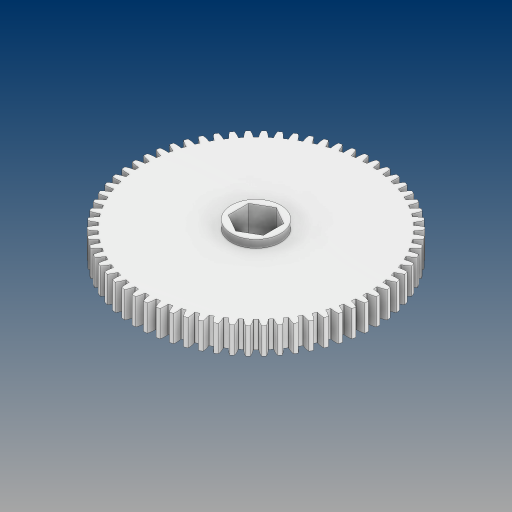
# Autodesk Inventor part: SHOT_1_004_66TGear-24TPulley
Saved by Autodesk Inventor 2024.3 (Build 283343000, 343)
## iProperties
Created: 2024-08-09
Part Number: SHOT_1_004_66TGear-24TPulley
Material: ABS Plastic
Document SubType Name: Modeling
Designer: Kenji
Density: 1.06 g/cm^3
Appearance: Smooth - White
Author: Kenji
Autodesk Inventor part; units mm, degrees
(part 1 of 2)
ref_plane "YZ Plane" through (0, 0, 0) normal (1, 0, 0) x (0, 1, 0)
ref_plane "XZ Plane" through (0, 0, 0) normal (0, 1, 0) x (-1, 0, 0)
ref_plane "XY Plane" through (0, 0, 0) normal (0, 0, 1) x (1, 0, 0)
sketch "Sketch1" plane through (0, 0, 0) normal (0, 1, 0) x (-1, 0, 0)
  circle A0 centre (0, 0) radius 41.91 construction
  line L0 (0, 0) -> (41.91, 0) construction
  line L1 (0, 0) -> (39.2827, 10.1592) construction
  line L2 (39.2827, 10.1592) -> (41.91, 0) construction
  arc A1 (39.2827, 10.1592) -> (37.9956, 14.2362) centre (0, 0) ccw construction
  arc A2 (40.5744, -0.225) -> (39.2827, 10.1592) centre (0, 0) ccw construction
  circle A3 centre (0, 0) radius 43.18
  line L3 (40.3225, 15.447) -> (40.3225, -15.447) construction
  line L4 (40.5744, -0.225) -> (41.91, 0) construction
  line L5 (40.5744, -0.225) -> (40.3225, -0.2901) construction
  line L6 (41.4814, 11.992) -> (38.8764, -18.7919) construction
  line L7 (40.5744, -0.225) -> (40.4457, -0.2469) construction
  line L8 (40.4457, -0.2469) -> (40.3225, -0.2901) construction
  line L9 (41.6879, 11.253) -> (38.5364, -19.4798) construction
  line L10 (40.5744, -0.225) -> (40.5099, -0.2348) construction
  line L11 (40.5099, -0.2348) -> (40.4457, -0.2469) construction
  line L12 (41.1912, 12.9537) -> (39.303, -17.8825) construction
  line L13 (40.5744, -0.225) -> (40.382, -0.2624) construction
  line L14 (40.4457, -0.2469) -> (40.382, -0.2624) construction
  line L15 (40.382, -0.2624) -> (40.3225, -0.2901) construction
  spline S0 degree 4 poles (40.5744, -0.225) (40.5088, -0.2321) (40.4478, -0.2504) (40.3776, -0.2514) (40.3225, -0.2901) knots 0 0 0 0 0 1 1 1 1 1
  line L16 (37.9956, 14.2362) -> (43.1781, 0.4045) construction
  arc A4 (40.3121, -0.9596) -> (40.3225, -0.2901) centre (0, 0) ccw
  line L17 (40.3121, -0.9596) -> (0, 0) construction
  arc A5 (43.1678, -1.0276) -> (43.1781, 0.4045) centre (0, 0) ccw construction
  line L18 (43.1678, -1.0276) -> (40.3121, -0.9596) construction
  arc A6 (43.11, -2.4585) -> (43.1678, -1.0276) centre (0, 0) ccw construction
  spline S1 degree 2 poles (43.1781, 0.4045) (41.9324, -0.0925) (40.5744, -0.225) knots 0 0 0 1 1 1
  spline S2 degree 4 poles (40.5392, -1.7059) (40.4739, -1.6957) (40.4139, -1.6745) (40.3438, -1.6702) (40.2906, -1.6288) knots 0 0 0 0 0 1 1 1 1 1
  arc A7 (40.2906, -1.6288) -> (40.3121, -0.9596) centre (0, 0) ccw
  spline S3 degree 2 poles (43.11, -2.4585) (41.8893, -1.9028) (40.5392, -1.7059) knots 0 0 0 1 1 1
  spline S4 degree 2 poles (42.9441, 4.507) (41.7513, 3.8939) (40.4121, 3.6329) knots 0 0 0 1 1 1
  spline S5 degree 2 poles (43.1484, 1.6505) (41.8805, 2.0876) (40.5178, 2.1553) knots 0 0 0 1 1 1
  spline S6 degree 4 poles (40.5178, 2.1553) (40.4519, 2.1593) (40.39, 2.1747) (40.3199, 2.1723) (40.263, 2.2084) knots 0 0 0 0 0 1 1 1 1 1
  arc A8 (40.263, 2.2084) -> (40.2208, 2.8766) centre (0, 0) ccw
  arc A9 (40.2208, 2.8766) -> (40.1675, 3.5441) centre (0, 0) ccw
  spline S7 degree 4 poles (40.4121, 3.6329) (40.3474, 3.6196) (40.2884, 3.5956) (40.2187, 3.5879) (40.1675, 3.5441) knots 0 0 0 0 0 1 1 1 1 1
  spline S8 degree 2 poles (42.3213, 8.5687) (41.1921, 7.845) (39.8838, 7.4578) knots 0 0 0 1 1 1
  spline S9 degree 2 poles (42.7962, 5.7445) (41.4924, 6.0591) (40.1294, 5.997) knots 0 0 0 1 1 1
  spline S10 degree 4 poles (40.1294, 5.997) (40.0634, 5.9947) (40.0004, 6.0041) (39.9308, 5.9951) (39.8708, 6.0257) knots 0 0 0 0 0 1 1 1 1 1
  arc A10 (39.8708, 6.0257) -> (39.7652, 6.6869) centre (0, 0) ccw
  arc A11 (39.7652, 6.6869) -> (39.6487, 7.3462) centre (0, 0) ccw
  spline S11 degree 4 poles (39.8838, 7.4578) (39.8207, 7.4385) (39.7642, 7.409) (39.6955, 7.3947) (39.6487, 7.3462) knots 0 0 0 0 0 1 1 1 1 1
  spline S12 degree 2 poles (41.3151, 12.5528) (40.2599, 11.725) (38.9943, 11.2153) knots 0 0 0 1 1 1
  spline S13 degree 2 poles (42.0563, 9.7866) (40.7286, 9.9758) (39.3777, 9.7844) knots 0 0 0 1 1 1
  spline S14 degree 4 poles (39.3777, 9.7844) (39.3122, 9.7758) (39.2486, 9.7792) (39.1802, 9.7636) (39.1175, 9.7883) knots 0 0 0 0 0 1 1 1 1 1
  arc A12 (39.1175, 9.7883) -> (38.9496, 10.4365) centre (0, 0) ccw
  arc A13 (38.9496, 10.4365) -> (38.7709, 11.0818) centre (0, 0) ccw
  spline S15 degree 4 poles (38.9943, 11.2153) (38.9333, 11.19) (38.8799, 11.1552) (38.8128, 11.1345) (38.7709, 11.0818) knots 0 0 0 0 0 1 1 1 1 1
  spline S16 degree 2 poles (39.9348, 16.4232) (38.9631, 15.4988) (37.7516, 14.8711) knots 0 0 0 1 1 1
  spline S17 degree 2 poles (40.9356, 13.7399) (39.5959, 13.8021) (38.2693, 13.4832) knots 0 0 0 1 1 1
  spline S18 degree 4 poles (38.2693, 13.4832) (38.2049, 13.4684) (38.1413, 13.4658) (38.0746, 13.4437) (38.0099, 13.4624) knots 0 0 0 0 0 1 1 1 1 1
  arc A14 (38.0099, 13.4624) -> (37.7811, 14.0916) centre (0, 0) ccw
  arc A15 (37.7811, 14.0916) -> (37.5419, 14.717) centre (0, 0) ccw
  spline S19 degree 4 poles (37.7516, 14.8711) (37.6933, 14.8402) (37.6434, 14.8005) (37.5787, 14.7735) (37.5419, 14.717) knots 0 0 0 0 0 1 1 1 1 1
  spline S20 degree 2 poles (38.1929, 20.1449) (37.3134, 19.1323) (36.1671, 18.3923) knots 0 0 0 1 1 1
  spline S21 degree 2 poles (39.4442, 17.5689) (38.1047, 17.5035) (36.8144, 17.0599) knots 0 0 0 1 1 1
  spline S22 degree 4 poles (36.8144, 17.0599) (36.7517, 17.039) (36.6886, 17.0303) (36.6243, 17.0021) (36.5581, 17.0145) knots 0 0 0 0 0 1 1 1 1 1
  arc A16 (36.5581, 17.0145) -> (36.2706, 17.6192) centre (0, 0) ccw
  arc A17 (36.2706, 17.6192) -> (35.973, 18.219) centre (0, 0) ccw
  spline S23 degree 4 poles (36.1671, 18.3923) (36.112, 18.3559) (36.0661, 18.3117) (36.0042, 18.2787) (35.973, 18.219) knots 0 0 0 0 0 1 1 1 1 1
  spline S24 degree 2 poles (36.1051, 23.6841) (35.3258, 22.5926) (34.255, 21.7469) knots 0 0 0 1 1 1
  spline S25 degree 2 poles (37.5956, 21.2388) (36.2683, 21.0463) (35.026, 20.4821) knots 0 0 0 1 1 1
  spline S26 degree 4 poles (35.026, 20.4821) (34.9656, 20.4554) (34.9036, 20.4407) (34.8423, 20.4065) (34.7752, 20.4125) knots 0 0 0 0 0 1 1 1 1 1
  arc A18 (34.7752, 20.4125) -> (34.4315, 20.9871) centre (0, 0) ccw
  arc A19 (34.4315, 20.9871) -> (34.0783, 21.5559) centre (0, 0) ccw
  spline S27 degree 4 poles (34.255, 21.7469) (34.2036, 21.7055) (34.1622, 21.6571) (34.1037, 21.6183) (34.0783, 21.5559) knots 0 0 0 0 0 1 1 1 1 1
  spline S28 degree 2 poles (33.6903, 27.0089) (33.0183, 25.8482) (32.0327, 24.9046) knots 0 0 0 1 1 1
  spline S29 degree 2 poles (35.4065, 24.7163) (34.1035, 24.3985) (32.9205, 23.7188) knots 0 0 0 1 1 1
  spline S30 degree 4 poles (32.9205, 23.7188) (32.8629, 23.6864) (32.8026, 23.6659) (32.7448, 23.626) (32.6774, 23.6257) knots 0 0 0 0 0 1 1 1 1 1
  arc A20 (32.6774, 23.6257) -> (32.2807, 24.165) centre (0, 0) ccw
  arc A21 (32.2807, 24.165) -> (31.875, 24.6977) centre (0, 0) ccw
  spline S31 degree 4 poles (32.0327, 24.9046) (31.9855, 24.8585) (31.9488, 24.8064) (31.8943, 24.7622) (31.875, 24.6977) knots 0 0 0 0 0 1 1 1 1 1
  spline S32 degree 2 poles (30.9703, 30.089) (30.4117, 28.8697) (29.5204, 27.8367) knots 0 0 0 1 1 1
  spline S33 degree 2 poles (32.8967, 27.97) (31.6298, 27.5298) (30.5168, 26.7406) knots 0 0 0 1 1 1
  spline S34 degree 4 poles (30.5168, 26.7406) (30.4625, 26.703) (30.4044, 26.6769) (30.3507, 26.6317) (30.2837, 26.6249) knots 0 0 0 0 0 1 1 1 1 1
  arc A22 (30.2837, 26.6249) -> (29.8375, 27.1241) centre (0, 0) ccw
  arc A23 (29.8375, 27.1241) -> (29.383, 27.6157) centre (0, 0) ccw
  spline S35 degree 4 poles (29.5204, 27.8367) (29.4777, 27.7863) (29.4462, 27.731) (29.3961, 27.6818) (29.383, 27.6157) knots 0 0 0 0 0 1 1 1 1 1
  spline S36 degree 2 poles (27.97, 32.8967) (27.5298, 31.6298) (26.7406, 30.5168) knots 0 0 0 1 1 1
  spline S37 degree 2 poles (30.089, 30.9703) (28.8697, 30.4117) (27.8367, 29.5204) knots 0 0 0 1 1 1
  spline S38 degree 4 poles (27.8367, 29.5204) (27.7863, 29.4777) (27.731, 29.4462) (27.6818, 29.3961) (27.6157, 29.383) knots 0 0 0 0 0 1 1 1 1 1
  arc A24 (27.6157, 29.383) -> (27.1241, 29.8375) centre (0, 0) ccw
  arc A25 (27.1241, 29.8375) -> (26.6249, 30.2837) centre (0, 0) ccw
  spline S39 degree 4 poles (26.7406, 30.5168) (26.703, 30.4625) (26.6769, 30.4044) (26.6317, 30.3507) (26.6249, 30.2837) knots 0 0 0 0 0 1 1 1 1 1
  spline S40 degree 2 poles (24.7163, 35.4065) (24.3985, 34.1035) (23.7188, 32.9205) knots 0 0 0 1 1 1
  spline S41 degree 2 poles (27.0089, 33.6903) (25.8482, 33.0183) (24.9046, 32.0327) knots 0 0 0 1 1 1
  spline S42 degree 4 poles (24.9046, 32.0327) (24.8585, 31.9855) (24.8064, 31.9488) (24.7622, 31.8943) (24.6977, 31.875) knots 0 0 0 0 0 1 1 1 1 1
  arc A26 (24.6977, 31.875) -> (24.165, 32.2807) centre (0, 0) ccw
  arc A27 (24.165, 32.2807) -> (23.6257, 32.6774) centre (0, 0) ccw
  spline S43 degree 4 poles (23.7188, 32.9205) (23.6864, 32.8629) (23.6659, 32.8026) (23.626, 32.7448) (23.6257, 32.6774) knots 0 0 0 0 0 1 1 1 1 1
  spline S44 degree 2 poles (21.2388, 37.5956) (21.0463, 36.2683) (20.4821, 35.026) knots 0 0 0 1 1 1
  spline S45 degree 2 poles (23.6841, 36.1051) (22.5926, 35.3258) (21.7469, 34.255) knots 0 0 0 1 1 1
  spline S46 degree 4 poles (21.7469, 34.255) (21.7055, 34.2036) (21.6571, 34.1622) (21.6183, 34.1037) (21.5559, 34.0783) knots 0 0 0 0 0 1 1 1 1 1
  arc A28 (21.5559, 34.0783) -> (20.9871, 34.4315) centre (0, 0) ccw
  arc A29 (20.9871, 34.4315) -> (20.4125, 34.7752) centre (0, 0) ccw
  spline S47 degree 4 poles (20.4821, 35.026) (20.4554, 34.9656) (20.4407, 34.9036) (20.4065, 34.8423) (20.4125, 34.7752) knots 0 0 0 0 0 1 1 1 1 1
  spline S48 degree 2 poles (17.5689, 39.4442) (17.5035, 38.1047) (17.0599, 36.8144) knots 0 0 0 1 1 1
  spline S49 degree 2 poles (20.1449, 38.1929) (19.1323, 37.3134) (18.3923, 36.1671) knots 0 0 0 1 1 1
  spline S50 degree 4 poles (18.3923, 36.1671) (18.3559, 36.112) (18.3117, 36.0661) (18.2787, 36.0042) (18.219, 35.973) knots 0 0 0 0 0 1 1 1 1 1
  arc A30 (18.219, 35.973) -> (17.6192, 36.2706) centre (0, 0) ccw
  arc A31 (17.6192, 36.2706) -> (17.0145, 36.5581) centre (0, 0) ccw
  spline S51 degree 4 poles (17.0599, 36.8144) (17.039, 36.7517) (17.0303, 36.6886) (17.0021, 36.6243) (17.0145, 36.5581) knots 0 0 0 0 0 1 1 1 1 1
  spline S52 degree 2 poles (13.7399, 40.9356) (13.8021, 39.5959) (13.4832, 38.2693) knots 0 0 0 1 1 1
  spline S53 degree 2 poles (16.4232, 39.9348) (15.4988, 38.9631) (14.8711, 37.7516) knots 0 0 0 1 1 1
  spline S54 degree 4 poles (14.8711, 37.7516) (14.8402, 37.6933) (14.8005, 37.6434) (14.7735, 37.5787) (14.717, 37.5419) knots 0 0 0 0 0 1 1 1 1 1
  arc A32 (14.717, 37.5419) -> (14.0916, 37.7811) centre (0, 0) ccw
  arc A33 (14.0916, 37.7811) -> (13.4624, 38.0099) centre (0, 0) ccw
  spline S55 degree 4 poles (13.4832, 38.2693) (13.4684, 38.2049) (13.4658, 38.1413) (13.4437, 38.0746) (13.4624, 38.0099) knots 0 0 0 0 0 1 1 1 1 1
  spline S56 degree 2 poles (9.7866, 42.0563) (9.9758, 40.7286) (9.7844, 39.3777) knots 0 0 0 1 1 1
  spline S57 degree 2 poles (12.5528, 41.3151) (11.725, 40.2599) (11.2153, 38.9943) knots 0 0 0 1 1 1
  spline S58 degree 4 poles (11.2153, 38.9943) (11.19, 38.9333) (11.1552, 38.8799) (11.1345, 38.8128) (11.0818, 38.7709) knots 0 0 0 0 0 1 1 1 1 1
  arc A34 (11.0818, 38.7709) -> (10.4365, 38.9496) centre (0, 0) ccw
  arc A35 (10.4365, 38.9496) -> (9.7883, 39.1175) centre (0, 0) ccw
  spline S59 degree 4 poles (9.7844, 39.3777) (9.7758, 39.3122) (9.7792, 39.2486) (9.7636, 39.1802) (9.7883, 39.1175) knots 0 0 0 0 0 1 1 1 1 1
  spline S60 degree 2 poles (5.7445, 42.7962) (6.0591, 41.4924) (5.997, 40.1294) knots 0 0 0 1 1 1
  spline S61 degree 2 poles (8.5687, 42.3213) (7.845, 41.1921) (7.4578, 39.8838) knots 0 0 0 1 1 1
  spline S62 degree 4 poles (7.4578, 39.8838) (7.4385, 39.8207) (7.409, 39.7642) (7.3947, 39.6955) (7.3462, 39.6487) knots 0 0 0 0 0 1 1 1 1 1
  arc A36 (7.3462, 39.6487) -> (6.6869, 39.7652) centre (0, 0) ccw
  arc A37 (6.6869, 39.7652) -> (6.0257, 39.8708) centre (0, 0) ccw
  spline S63 degree 4 poles (5.997, 40.1294) (5.9947, 40.0634) (6.0041, 40.0004) (5.9951, 39.9308) (6.0257, 39.8708) knots 0 0 0 0 0 1 1 1 1 1
  spline S64 degree 2 poles (1.6505, 43.1484) (2.0876, 41.8805) (2.1553, 40.5178) knots 0 0 0 1 1 1
  spline S65 degree 2 poles (4.507, 42.9441) (3.8939, 41.7513) (3.6329, 40.4121) knots 0 0 0 1 1 1
  spline S66 degree 4 poles (3.6329, 40.4121) (3.6196, 40.3474) (3.5956, 40.2884) (3.5879, 40.2187) (3.5441, 40.1675) knots 0 0 0 0 0 1 1 1 1 1
  arc A38 (3.5441, 40.1675) -> (2.8766, 40.2208) centre (0, 0) ccw
  arc A39 (2.8766, 40.2208) -> (2.2084, 40.263) centre (0, 0) ccw
  spline S67 degree 4 poles (2.1553, 40.5178) (2.1593, 40.4519) (2.1747, 40.39) (2.1723, 40.3199) (2.2084, 40.263) knots 0 0 0 0 0 1 1 1 1 1
  spline S68 degree 2 poles (-2.4585, 43.11) (-1.9028, 41.8893) (-1.7059, 40.5392) knots 0 0 0 1 1 1
  spline S69 degree 2 poles (0.4045, 43.1781) (-0.0925, 41.9324) (-0.225, 40.5744) knots 0 0 0 1 1 1
  spline S70 degree 4 poles (-0.225, 40.5744) (-0.2321, 40.5088) (-0.2504, 40.4478) (-0.2514, 40.3776) (-0.2901, 40.3225) knots 0 0 0 0 0 1 1 1 1 1
  arc A40 (-0.2901, 40.3225) -> (-0.9596, 40.3121) centre (0, 0) ccw
  arc A41 (-0.9596, 40.3121) -> (-1.6288, 40.2906) centre (0, 0) ccw
  spline S71 degree 4 poles (-1.7059, 40.5392) (-1.6957, 40.4739) (-1.6745, 40.4139) (-1.6702, 40.3438) (-1.6288, 40.2906) knots 0 0 0 0 0 1 1 1 1 1
  spline S72 degree 2 poles (-6.5452, 42.6811) (-5.8761, 41.5188) (-5.5517, 40.1935) knots 0 0 0 1 1 1
  spline S73 degree 2 poles (-3.7017, 43.021) (-4.078, 41.7338) (-4.0808, 40.3693) knots 0 0 0 1 1 1
  spline S74 degree 4 poles (-4.0808, 40.3693) (-4.0816, 40.3033) (-4.094, 40.2408) (-4.0883, 40.1709) (-4.1217, 40.1123) knots 0 0 0 0 0 1 1 1 1 1
  arc A42 (-4.1217, 40.1123) -> (-4.7872, 40.0384) centre (0, 0) ccw
  arc A43 (-4.7872, 40.0384) -> (-5.4513, 39.9534) centre (0, 0) ccw
  spline S75 degree 4 poles (-5.5517, 40.1935) (-5.5353, 40.1295) (-5.5085, 40.0717) (-5.4975, 40.0024) (-5.4513, 39.9534) knots 0 0 0 0 0 1 1 1 1 1
  spline S76 degree 2 poles (-10.5727, 41.8656) (-9.7961, 40.7722) (-9.3471, 39.4838) knots 0 0 0 1 1 1
  spline S77 degree 2 poles (-7.7743, 42.4744) (-8.0266, 41.1571) (-7.8997, 39.7986) knots 0 0 0 1 1 1
  spline S78 degree 4 poles (-7.8997, 39.7986) (-7.8942, 39.7328) (-7.9006, 39.6694) (-7.8883, 39.6003) (-7.916, 39.5389) knots 0 0 0 0 0 1 1 1 1 1
  arc A44 (-7.916, 39.5389) -> (-8.5714, 39.402) centre (0, 0) ccw
  arc A45 (-8.5714, 39.402) -> (-9.2244, 39.2543) centre (0, 0) ccw
  spline S79 degree 4 poles (-9.3471, 39.4838) (-9.3248, 39.4216) (-9.2926, 39.3666) (-9.2751, 39.2987) (-9.2244, 39.2543) knots 0 0 0 0 0 1 1 1 1 1
  spline S80 degree 2 poles (-14.5044, 40.6711) (-13.6274, 39.6564) (-13.058, 38.4165) knots 0 0 0 1 1 1
  spline S81 degree 2 poles (-11.7766, 41.543) (-11.9025, 40.2078) (-11.647, 38.8675) knots 0 0 0 1 1 1
  spline S82 degree 4 poles (-11.647, 38.8675) (-11.6353, 38.8025) (-11.6357, 38.7388) (-11.6169, 38.6712) (-11.6385, 38.6074) knots 0 0 0 0 0 1 1 1 1 1
  arc A46 (-11.6385, 38.6074) -> (-12.278, 38.4088) centre (0, 0) ccw
  arc A47 (-12.278, 38.4088) -> (-12.914, 38.1997) centre (0, 0) ccw
  spline S83 degree 4 poles (-13.058, 38.4165) (-13.0298, 38.3567) (-12.9926, 38.305) (-12.9687, 38.2391) (-12.914, 38.1997) knots 0 0 0 0 0 1 1 1 1 1
  spline S84 degree 2 poles (-18.3048, 39.1082) (-17.3352, 38.1815) (-16.6506, 37.0013) knots 0 0 0 1 1 1
  spline S85 degree 2 poles (-15.6722, 40.2355) (-15.6706, 38.8943) (-15.2889, 37.5844) knots 0 0 0 1 1 1
  spline S86 degree 4 poles (-15.2889, 37.5844) (-15.271, 37.5208) (-15.2653, 37.4574) (-15.2402, 37.3918) (-15.2557, 37.3263) knots 0 0 0 0 0 1 1 1 1 1
  arc A48 (-15.2557, 37.3263) -> (-15.8734, 37.0678) centre (0, 0) ccw
  arc A49 (-15.8734, 37.0678) -> (-16.4867, 36.7992) centre (0, 0) ccw
  spline S87 degree 4 poles (-16.6506, 37.0013) (-16.6169, 36.9445) (-16.5749, 36.8966) (-16.5448, 36.8332) (-16.4867, 36.7992) knots 0 0 0 0 0 1 1 1 1 1
  spline S88 degree 2 poles (-21.9393, 37.1911) (-20.8861, 36.3608) (-20.0924, 35.251) knots 0 0 0 1 1 1
  spline S89 degree 2 poles (-19.4258, 38.5636) (-19.2967, 37.2286) (-18.7923, 35.9609) knots 0 0 0 1 1 1
  spline S90 degree 4 poles (-18.7923, 35.9609) (-18.7685, 35.8993) (-18.7568, 35.8367) (-18.7255, 35.7739) (-18.7347, 35.7071) knots 0 0 0 0 0 1 1 1 1 1
  arc A50 (-18.7347, 35.7071) -> (-19.325, 35.3911) centre (0, 0) ccw
  arc A51 (-19.325, 35.3911) -> (-19.91, 35.0654) centre (0, 0) ccw
  spline S91 degree 4 poles (-20.0924, 35.251) (-20.0534, 35.1977) (-20.0071, 35.154) (-19.9711, 35.0937) (-19.91, 35.0654) knots 0 0 0 0 0 1 1 1 1 1
  spline S92 degree 2 poles (-25.3752, 34.9372) (-24.2479, 34.2108) (-23.3522, 33.1815) knots 0 0 0 1 1 1
  spline S93 degree 2 poles (-23.0036, 36.5424) (-22.7482, 35.2258) (-22.1255, 34.0118) knots 0 0 0 1 1 1
  spline S94 degree 4 poles (-22.1255, 34.0118) (-22.0959, 33.9527) (-22.0783, 33.8915) (-22.0412, 33.8319) (-22.0441, 33.7646) knots 0 0 0 0 0 1 1 1 1 1
  arc A52 (-22.0441, 33.7646) -> (-22.6017, 33.3939) centre (0, 0) ccw
  arc A53 (-22.6017, 33.3939) -> (-23.153, 33.014) centre (0, 0) ccw
  spline S95 degree 4 poles (-23.3522, 33.1815) (-23.3084, 33.1321) (-23.2581, 33.093) (-23.2166, 33.0364) (-23.153, 33.014) knots 0 0 0 0 0 1 1 1 1 1
  spline S96 degree 2 poles (-28.5813, 32.367) (-27.39, 31.751) (-26.4006, 30.8115) knots 0 0 0 1 1 1
  spline S97 degree 2 poles (-26.373, 34.1903) (-25.9936, 32.9039) (-25.2583, 31.7546) knots 0 0 0 1 1 1
  spline S98 degree 4 poles (-25.2583, 31.7546) (-25.2233, 31.6986) (-25.1999, 31.6393) (-25.1573, 31.5836) (-25.1538, 31.5163) knots 0 0 0 0 0 1 1 1 1 1
  arc A54 (-25.1538, 31.5163) -> (-25.6736, 31.0943) centre (0, 0) ccw
  arc A55 (-25.6736, 31.0943) -> (-26.1864, 30.6637) centre (0, 0) ccw
  spline S99 degree 4 poles (-26.4006, 30.8115) (-26.3522, 30.7665) (-26.2984, 30.7323) (-26.2517, 30.6799) (-26.1864, 30.6637) knots 0 0 0 0 0 1 1 1 1 1
  spline S100 degree 2 poles (-31.5286, 29.5036) (-30.2841, 29.0036) (-29.2099, 28.1624) knots 0 0 0 1 1 1
  spline S101 degree 2 poles (-29.5036, 31.5286) (-29.0036, 30.2841) (-28.1624, 29.2099) knots 0 0 0 1 1 1
  spline S102 degree 4 poles (-28.1624, 29.2099) (-28.1222, 29.1574) (-28.0933, 29.1007) (-28.0456, 29.0492) (-28.0357, 28.9825) knots 0 0 0 0 0 1 1 1 1 1
  arc A56 (-28.0357, 28.9825) -> (-28.5131, 28.5131) centre (0, 0) ccw
  arc A57 (-28.5131, 28.5131) -> (-28.9825, 28.0357) centre (0, 0) ccw
  spline S103 degree 4 poles (-29.2099, 28.1624) (-29.1574, 28.1222) (-29.1007, 28.0933) (-29.0492, 28.0456) (-28.9825, 28.0357) knots 0 0 0 0 0 1 1 1 1 1
  spline S104 degree 2 poles (-34.1903, 26.373) (-32.9039, 25.9936) (-31.7546, 25.2583) knots 0 0 0 1 1 1
  spline S105 degree 2 poles (-32.367, 28.5813) (-31.751, 27.39) (-30.8115, 26.4006) knots 0 0 0 1 1 1
  spline S106 degree 4 poles (-30.8115, 26.4006) (-30.7665, 26.3522) (-30.7323, 26.2984) (-30.6799, 26.2517) (-30.6637, 26.1864) knots 0 0 0 0 0 1 1 1 1 1
  arc A58 (-30.6637, 26.1864) -> (-31.0943, 25.6736) centre (0, 0) ccw
  arc A59 (-31.0943, 25.6736) -> (-31.5163, 25.1538) centre (0, 0) ccw
  spline S107 degree 4 poles (-31.7546, 25.2583) (-31.6986, 25.2233) (-31.6393, 25.1999) (-31.5836, 25.1573) (-31.5163, 25.1538) knots 0 0 0 0 0 1 1 1 1 1
  spline S108 degree 2 poles (-36.5424, 23.0036) (-35.2258, 22.7482) (-34.0118, 22.1255) knots 0 0 0 1 1 1
  spline S109 degree 2 poles (-34.9372, 25.3752) (-34.2108, 24.2479) (-33.1815, 23.3522) knots 0 0 0 1 1 1
  spline S110 degree 4 poles (-33.1815, 23.3522) (-33.1321, 23.3084) (-33.093, 23.2581) (-33.0364, 23.2166) (-33.014, 23.153) knots 0 0 0 0 0 1 1 1 1 1
  arc A60 (-33.014, 23.153) -> (-33.3939, 22.6017) centre (0, 0) ccw
  arc A61 (-33.3939, 22.6017) -> (-33.7646, 22.0441) centre (0, 0) ccw
  spline S111 degree 4 poles (-34.0118, 22.1255) (-33.9527, 22.0959) (-33.8915, 22.0783) (-33.8319, 22.0412) (-33.7646, 22.0441) knots 0 0 0 0 0 1 1 1 1 1
  spline S112 degree 2 poles (-38.5636, 19.4258) (-37.2286, 19.2967) (-35.9609, 18.7923) knots 0 0 0 1 1 1
  spline S113 degree 2 poles (-37.1911, 21.9393) (-36.3608, 20.8861) (-35.251, 20.0924) knots 0 0 0 1 1 1
  spline S114 degree 4 poles (-35.251, 20.0924) (-35.1977, 20.0534) (-35.154, 20.0071) (-35.0937, 19.9711) (-35.0654, 19.91) knots 0 0 0 0 0 1 1 1 1 1
  arc A62 (-35.0654, 19.91) -> (-35.3911, 19.325) centre (0, 0) ccw
  arc A63 (-35.3911, 19.325) -> (-35.7071, 18.7347) centre (0, 0) ccw
  spline S115 degree 4 poles (-35.9609, 18.7923) (-35.8993, 18.7685) (-35.8367, 18.7568) (-35.7739, 18.7255) (-35.7071, 18.7347) knots 0 0 0 0 0 1 1 1 1 1
  spline S116 degree 2 poles (-40.2355, 15.6722) (-38.8943, 15.6706) (-37.5844, 15.2889) knots 0 0 0 1 1 1
  spline S117 degree 2 poles (-39.1082, 18.3048) (-38.1815, 17.3352) (-37.0013, 16.6506) knots 0 0 0 1 1 1
  spline S118 degree 4 poles (-37.0013, 16.6506) (-36.9445, 16.6169) (-36.8966, 16.5749) (-36.8332, 16.5448) (-36.7992, 16.4867) knots 0 0 0 0 0 1 1 1 1 1
  arc A64 (-36.7992, 16.4867) -> (-37.0678, 15.8734) centre (0, 0) ccw
  arc A65 (-37.0678, 15.8734) -> (-37.3263, 15.2557) centre (0, 0) ccw
  spline S119 degree 4 poles (-37.5844, 15.2889) (-37.5208, 15.271) (-37.4574, 15.2653) (-37.3918, 15.2402) (-37.3263, 15.2557) knots 0 0 0 0 0 1 1 1 1 1
  spline S120 degree 2 poles (-41.543, 11.7766) (-40.2078, 11.9025) (-38.8675, 11.647) knots 0 0 0 1 1 1
  spline S121 degree 2 poles (-40.6711, 14.5044) (-39.6564, 13.6274) (-38.4165, 13.058) knots 0 0 0 1 1 1
  spline S122 degree 4 poles (-38.4165, 13.058) (-38.3567, 13.0298) (-38.305, 12.9926) (-38.2391, 12.9687) (-38.1997, 12.914) knots 0 0 0 0 0 1 1 1 1 1
  arc A66 (-38.1997, 12.914) -> (-38.4088, 12.278) centre (0, 0) ccw
  arc A67 (-38.4088, 12.278) -> (-38.6074, 11.6385) centre (0, 0) ccw
  spline S123 degree 4 poles (-38.8675, 11.647) (-38.8025, 11.6353) (-38.7388, 11.6357) (-38.6712, 11.6169) (-38.6074, 11.6385) knots 0 0 0 0 0 1 1 1 1 1
  spline S124 degree 2 poles (-42.4744, 7.7743) (-41.1571, 8.0266) (-39.7986, 7.8997) knots 0 0 0 1 1 1
  spline S125 degree 2 poles (-41.8656, 10.5727) (-40.7722, 9.7961) (-39.4838, 9.3471) knots 0 0 0 1 1 1
  spline S126 degree 4 poles (-39.4838, 9.3471) (-39.4216, 9.3248) (-39.3666, 9.2926) (-39.2987, 9.2751) (-39.2543, 9.2244) knots 0 0 0 0 0 1 1 1 1 1
  arc A68 (-39.2543, 9.2244) -> (-39.402, 8.5714) centre (0, 0) ccw
  arc A69 (-39.402, 8.5714) -> (-39.5389, 7.916) centre (0, 0) ccw
  spline S127 degree 4 poles (-39.7986, 7.8997) (-39.7328, 7.8942) (-39.6694, 7.9006) (-39.6003, 7.8883) (-39.5389, 7.916) knots 0 0 0 0 0 1 1 1 1 1
  spline S128 degree 2 poles (-43.021, 3.7017) (-41.7338, 4.078) (-40.3693, 4.0808) knots 0 0 0 1 1 1
  spline S129 degree 2 poles (-42.6811, 6.5452) (-41.5188, 5.8761) (-40.1935, 5.5517) knots 0 0 0 1 1 1
  spline S130 degree 4 poles (-40.1935, 5.5517) (-40.1295, 5.5353) (-40.0717, 5.5085) (-40.0024, 5.4975) (-39.9534, 5.4513) knots 0 0 0 0 0 1 1 1 1 1
  arc A70 (-39.9534, 5.4513) -> (-40.0384, 4.7872) centre (0, 0) ccw
  arc A71 (-40.0384, 4.7872) -> (-40.1123, 4.1217) centre (0, 0) ccw
  spline S131 degree 4 poles (-40.3693, 4.0808) (-40.3033, 4.0816) (-40.2408, 4.094) (-40.1709, 4.0883) (-40.1123, 4.1217) knots 0 0 0 0 0 1 1 1 1 1
  spline S132 degree 2 poles (-43.1781, -0.4045) (-41.9324, 0.0925) (-40.5744, 0.225) knots 0 0 0 1 1 1
  spline S133 degree 2 poles (-43.11, 2.4585) (-41.8893, 1.9028) (-40.5392, 1.7059) knots 0 0 0 1 1 1
  spline S134 degree 4 poles (-40.5392, 1.7059) (-40.4739, 1.6957) (-40.4139, 1.6745) (-40.3438, 1.6702) (-40.2906, 1.6288) knots 0 0 0 0 0 1 1 1 1 1
  arc A72 (-40.2906, 1.6288) -> (-40.3121, 0.9596) centre (0, 0) ccw
  arc A73 (-40.3121, 0.9596) -> (-40.3225, 0.2901) centre (0, 0) ccw
  spline S135 degree 4 poles (-40.5744, 0.225) (-40.5088, 0.2321) (-40.4478, 0.2504) (-40.3776, 0.2514) (-40.3225, 0.2901) knots 0 0 0 0 0 1 1 1 1 1
  spline S136 degree 2 poles (-42.9441, -4.507) (-41.7513, -3.8939) (-40.4121, -3.6329) knots 0 0 0 1 1 1
  spline S137 degree 2 poles (-43.1484, -1.6505) (-41.8805, -2.0876) (-40.5178, -2.1553) knots 0 0 0 1 1 1
  spline S138 degree 4 poles (-40.5178, -2.1553) (-40.4519, -2.1593) (-40.39, -2.1747) (-40.3199, -2.1723) (-40.263, -2.2084) knots 0 0 0 0 0 1 1 1 1 1
  arc A74 (-40.263, -2.2084) -> (-40.2208, -2.8766) centre (0, 0) ccw
  arc A75 (-40.2208, -2.8766) -> (-40.1675, -3.5441) centre (0, 0) ccw
  spline S139 degree 4 poles (-40.4121, -3.6329) (-40.3474, -3.6196) (-40.2884, -3.5956) (-40.2187, -3.5879) (-40.1675, -3.5441) knots 0 0 0 0 0 1 1 1 1 1
  spline S140 degree 2 poles (-42.3213, -8.5687) (-41.1921, -7.845) (-39.8838, -7.4578) knots 0 0 0 1 1 1
  spline S141 degree 2 poles (-42.7962, -5.7445) (-41.4924, -6.0591) (-40.1294, -5.997) knots 0 0 0 1 1 1
  spline S142 degree 4 poles (-40.1294, -5.997) (-40.0634, -5.9947) (-40.0004, -6.0041) (-39.9308, -5.9951) (-39.8708, -6.0257) knots 0 0 0 0 0 1 1 1 1 1
  arc A76 (-39.8708, -6.0257) -> (-39.7652, -6.6869) centre (0, 0) ccw
  arc A77 (-39.7652, -6.6869) -> (-39.6487, -7.3462) centre (0, 0) ccw
  spline S143 degree 4 poles (-39.8838, -7.4578) (-39.8207, -7.4385) (-39.7642, -7.409) (-39.6955, -7.3947) (-39.6487, -7.3462) knots 0 0 0 0 0 1 1 1 1 1
  spline S144 degree 2 poles (-41.3151, -12.5528) (-40.2599, -11.725) (-38.9943, -11.2153) knots 0 0 0 1 1 1
  spline S145 degree 2 poles (-42.0563, -9.7866) (-40.7286, -9.9758) (-39.3777, -9.7844) knots 0 0 0 1 1 1
  spline S146 degree 4 poles (-39.3777, -9.7844) (-39.3122, -9.7758) (-39.2486, -9.7792) (-39.1802, -9.7636) (-39.1175, -9.7883) knots 0 0 0 0 0 1 1 1 1 1
  arc A78 (-39.1175, -9.7883) -> (-38.9496, -10.4365) centre (0, 0) ccw
  arc A79 (-38.9496, -10.4365) -> (-38.7709, -11.0818) centre (0, 0) ccw
  spline S147 degree 4 poles (-38.9943, -11.2153) (-38.9333, -11.19) (-38.8799, -11.1552) (-38.8128, -11.1345) (-38.7709, -11.0818) knots 0 0 0 0 0 1 1 1 1 1
  spline S148 degree 2 poles (-39.9348, -16.4232) (-38.9631, -15.4988) (-37.7516, -14.8711) knots 0 0 0 1 1 1
  spline S149 degree 2 poles (-40.9356, -13.7399) (-39.5959, -13.8021) (-38.2693, -13.4832) knots 0 0 0 1 1 1
  spline S150 degree 4 poles (-38.2693, -13.4832) (-38.2049, -13.4684) (-38.1413, -13.4658) (-38.0746, -13.4437) (-38.0099, -13.4624) knots 0 0 0 0 0 1 1 1 1 1
  arc A80 (-38.0099, -13.4624) -> (-37.7811, -14.0916) centre (0, 0) ccw
  arc A81 (-37.7811, -14.0916) -> (-37.5419, -14.717) centre (0, 0) ccw
  spline S151 degree 4 poles (-37.7516, -14.8711) (-37.6933, -14.8402) (-37.6434, -14.8005) (-37.5787, -14.7735) (-37.5419, -14.717) knots 0 0 0 0 0 1 1 1 1 1
  spline S152 degree 2 poles (-38.1929, -20.1449) (-37.3134, -19.1323) (-36.1671, -18.3923) knots 0 0 0 1 1 1
  spline S153 degree 2 poles (-39.4442, -17.5689) (-38.1047, -17.5035) (-36.8144, -17.0599) knots 0 0 0 1 1 1
  spline S154 degree 4 poles (-36.8144, -17.0599) (-36.7517, -17.039) (-36.6886, -17.0303) (-36.6243, -17.0021) (-36.5581, -17.0145) knots 0 0 0 0 0 1 1 1 1 1
  arc A82 (-36.5581, -17.0145) -> (-36.2706, -17.6192) centre (0, 0) ccw
  arc A83 (-36.2706, -17.6192) -> (-35.973, -18.219) centre (0, 0) ccw
  spline S155 degree 4 poles (-36.1671, -18.3923) (-36.112, -18.3559) (-36.0661, -18.3117) (-36.0042, -18.2787) (-35.973, -18.219) knots 0 0 0 0 0 1 1 1 1 1
  spline S156 degree 2 poles (-36.1051, -23.6841) (-35.3258, -22.5926) (-34.255, -21.7469) knots 0 0 0 1 1 1
  spline S157 degree 2 poles (-37.5956, -21.2388) (-36.2683, -21.0463) (-35.026, -20.4821) knots 0 0 0 1 1 1
  spline S158 degree 4 poles (-35.026, -20.4821) (-34.9656, -20.4554) (-34.9036, -20.4407) (-34.8423, -20.4065) (-34.7752, -20.4125) knots 0 0 0 0 0 1 1 1 1 1
  arc A84 (-34.7752, -20.4125) -> (-34.4315, -20.9871) centre (0, 0) ccw
  arc A85 (-34.4315, -20.9871) -> (-34.0783, -21.5559) centre (0, 0) ccw
  spline S159 degree 4 poles (-34.255, -21.7469) (-34.2036, -21.7055) (-34.1622, -21.6571) (-34.1037, -21.6183) (-34.0783, -21.5559) knots 0 0 0 0 0 1 1 1 1 1
  spline S160 degree 2 poles (-33.6903, -27.0089) (-33.0183, -25.8482) (-32.0327, -24.9046) knots 0 0 0 1 1 1
  spline S161 degree 2 poles (-35.4065, -24.7163) (-34.1035, -24.3985) (-32.9205, -23.7188) knots 0 0 0 1 1 1
  spline S162 degree 4 poles (-32.9205, -23.7188) (-32.8629, -23.6864) (-32.8026, -23.6659) (-32.7448, -23.626) (-32.6774, -23.6257) knots 0 0 0 0 0 1 1 1 1 1
  arc A86 (-32.6774, -23.6257) -> (-32.2807, -24.165) centre (0, 0) ccw
  arc A87 (-32.2807, -24.165) -> (-31.875, -24.6977) centre (0, 0) ccw
  spline S163 degree 4 poles (-32.0327, -24.9046) (-31.9855, -24.8585) (-31.9488, -24.8064) (-31.8943, -24.7622) (-31.875, -24.6977) knots 0 0 0 0 0 1 1 1 1 1
  spline S164 degree 2 poles (-30.9703, -30.089) (-30.4117, -28.8697) (-29.5204, -27.8367) knots 0 0 0 1 1 1
  spline S165 degree 2 poles (-32.8967, -27.97) (-31.6298, -27.5298) (-30.5168, -26.7406) knots 0 0 0 1 1 1
  spline S166 degree 4 poles (-30.5168, -26.7406) (-30.4625, -26.703) (-30.4044, -26.6769) (-30.3507, -26.6317) (-30.2837, -26.6249) knots 0 0 0 0 0 1 1 1 1 1
  arc A88 (-30.2837, -26.6249) -> (-29.8375, -27.1241) centre (0, 0) ccw
  arc A89 (-29.8375, -27.1241) -> (-29.383, -27.6157) centre (0, 0) ccw
  spline S167 degree 4 poles (-29.5204, -27.8367) (-29.4777, -27.7863) (-29.4462, -27.731) (-29.3961, -27.6818) (-29.383, -27.6157) knots 0 0 0 0 0 1 1 1 1 1
  spline S168 degree 2 poles (-27.97, -32.8967) (-27.5298, -31.6298) (-26.7406, -30.5168) knots 0 0 0 1 1 1
  spline S169 degree 2 poles (-30.089, -30.9703) (-28.8697, -30.4117) (-27.8367, -29.5204) knots 0 0 0 1 1 1
  spline S170 degree 4 poles (-27.8367, -29.5204) (-27.7863, -29.4777) (-27.731, -29.4462) (-27.6818, -29.3961) (-27.6157, -29.383) knots 0 0 0 0 0 1 1 1 1 1
  arc A90 (-27.6157, -29.383) -> (-27.1241, -29.8375) centre (0, 0) ccw
  arc A91 (-27.1241, -29.8375) -> (-26.6249, -30.2837) centre (0, 0) ccw
  spline S171 degree 4 poles (-26.7406, -30.5168) (-26.703, -30.4625) (-26.6769, -30.4044) (-26.6317, -30.3507) (-26.6249, -30.2837) knots 0 0 0 0 0 1 1 1 1 1
  spline S172 degree 2 poles (-24.7163, -35.4065) (-24.3985, -34.1035) (-23.7188, -32.9205) knots 0 0 0 1 1 1
  spline S173 degree 2 poles (-27.0089, -33.6903) (-25.8482, -33.0183) (-24.9046, -32.0327) knots 0 0 0 1 1 1
  spline S174 degree 4 poles (-24.9046, -32.0327) (-24.8585, -31.9855) (-24.8064, -31.9488) (-24.7622, -31.8943) (-24.6977, -31.875) knots 0 0 0 0 0 1 1 1 1 1
  arc A92 (-24.6977, -31.875) -> (-24.165, -32.2807) centre (0, 0) ccw
  arc A93 (-24.165, -32.2807) -> (-23.6257, -32.6774) centre (0, 0) ccw
  spline S175 degree 4 poles (-23.7188, -32.9205) (-23.6864, -32.8629) (-23.6659, -32.8026) (-23.626, -32.7448) (-23.6257, -32.6774) knots 0 0 0 0 0 1 1 1 1 1
  spline S176 degree 2 poles (-21.2388, -37.5956) (-21.0463, -36.2683) (-20.4821, -35.026) knots 0 0 0 1 1 1
  spline S177 degree 2 poles (-23.6841, -36.1051) (-22.5926, -35.3258) (-21.7469, -34.255) knots 0 0 0 1 1 1
  spline S178 degree 4 poles (-21.7469, -34.255) (-21.7055, -34.2036) (-21.6571, -34.1622) (-21.6183, -34.1037) (-21.5559, -34.0783) knots 0 0 0 0 0 1 1 1 1 1
  arc A94 (-21.5559, -34.0783) -> (-20.9871, -34.4315) centre (0, 0) ccw
  arc A95 (-20.9871, -34.4315) -> (-20.4125, -34.7752) centre (0, 0) ccw
  spline S179 degree 4 poles (-20.4821, -35.026) (-20.4554, -34.9656) (-20.4407, -34.9036) (-20.4065, -34.8423) (-20.4125, -34.7752) knots 0 0 0 0 0 1 1 1 1 1
  spline S180 degree 2 poles (-17.5689, -39.4442) (-17.5035, -38.1047) (-17.0599, -36.8144) knots 0 0 0 1 1 1
  spline S181 degree 2 poles (-20.1449, -38.1929) (-19.1323, -37.3134) (-18.3923, -36.1671) knots 0 0 0 1 1 1
  spline S182 degree 4 poles (-18.3923, -36.1671) (-18.3559, -36.112) (-18.3117, -36.0661) (-18.2787, -36.0042) (-18.219, -35.973) knots 0 0 0 0 0 1 1 1 1 1
  arc A96 (-18.219, -35.973) -> (-17.6192, -36.2706) centre (0, 0) ccw
  arc A97 (-17.6192, -36.2706) -> (-17.0145, -36.5581) centre (0, 0) ccw
  spline S183 degree 4 poles (-17.0599, -36.8144) (-17.039, -36.7517) (-17.0303, -36.6886) (-17.0021, -36.6243) (-17.0145, -36.5581) knots 0 0 0 0 0 1 1 1 1 1
  spline S184 degree 2 poles (-13.7399, -40.9356) (-13.8021, -39.5959) (-13.4832, -38.2693) knots 0 0 0 1 1 1
  spline S185 degree 2 poles (-16.4232, -39.9348) (-15.4988, -38.9631) (-14.8711, -37.7516) knots 0 0 0 1 1 1
  spline S186 degree 4 poles (-14.8711, -37.7516) (-14.8402, -37.6933) (-14.8005, -37.6434) (-14.7735, -37.5787) (-14.717, -37.5419) knots 0 0 0 0 0 1 1 1 1 1
  arc A98 (-14.717, -37.5419) -> (-14.0916, -37.7811) centre (0, 0) ccw
  arc A99 (-14.0916, -37.7811) -> (-13.4624, -38.0099) centre (0, 0) ccw
  spline S187 degree 4 poles (-13.4832, -38.2693) (-13.4684, -38.2049) (-13.4658, -38.1413) (-13.4437, -38.0746) (-13.4624, -38.0099) knots 0 0 0 0 0 1 1 1 1 1
  spline S188 degree 2 poles (-9.7866, -42.0563) (-9.9758, -40.7286) (-9.7844, -39.3777) knots 0 0 0 1 1 1
  spline S189 degree 2 poles (-12.5528, -41.3151) (-11.725, -40.2599) (-11.2153, -38.9943) knots 0 0 0 1 1 1
  spline S190 degree 4 poles (-11.2153, -38.9943) (-11.19, -38.9333) (-11.1552, -38.8799) (-11.1345, -38.8128) (-11.0818, -38.7709) knots 0 0 0 0 0 1 1 1 1 1
  arc A100 (-11.0818, -38.7709) -> (-10.4365, -38.9496) centre (0, 0) ccw
  arc A101 (-10.4365, -38.9496) -> (-9.7883, -39.1175) centre (0, 0) ccw
  spline S191 degree 4 poles (-9.7844, -39.3777) (-9.7758, -39.3122) (-9.7792, -39.2486) (-9.7636, -39.1802) (-9.7883, -39.1175) knots 0 0 0 0 0 1 1 1 1 1
  spline S192 degree 2 poles (-5.7445, -42.7962) (-6.0591, -41.4924) (-5.997, -40.1294) knots 0 0 0 1 1 1
  spline S193 degree 2 poles (-8.5687, -42.3213) (-7.845, -41.1921) (-7.4578, -39.8838) knots 0 0 0 1 1 1
  spline S194 degree 4 poles (-7.4578, -39.8838) (-7.4385, -39.8207) (-7.409, -39.7642) (-7.3947, -39.6955) (-7.3462, -39.6487) knots 0 0 0 0 0 1 1 1 1 1
  arc A102 (-7.3462, -39.6487) -> (-6.6869, -39.7652) centre (0, 0) ccw
  arc A103 (-6.6869, -39.7652) -> (-6.0257, -39.8708) centre (0, 0) ccw
  spline S195 degree 4 poles (-5.997, -40.1294) (-5.9947, -40.0634) (-6.0041, -40.0004) (-5.9951, -39.9308) (-6.0257, -39.8708) knots 0 0 0 0 0 1 1 1 1 1
  spline S196 degree 2 poles (-1.6505, -43.1484) (-2.0876, -41.8805) (-2.1553, -40.5178) knots 0 0 0 1 1 1
  spline S197 degree 2 poles (-4.507, -42.9441) (-3.8939, -41.7513) (-3.6329, -40.4121) knots 0 0 0 1 1 1
  spline S198 degree 4 poles (-3.6329, -40.4121) (-3.6196, -40.3474) (-3.5956, -40.2884) (-3.5879, -40.2187) (-3.5441, -40.1675) knots 0 0 0 0 0 1 1 1 1 1
  arc A104 (-3.5441, -40.1675) -> (-2.8766, -40.2208) centre (0, 0) ccw
  arc A105 (-2.8766, -40.2208) -> (-2.2084, -40.263) centre (0, 0) ccw
  spline S199 degree 4 poles (-2.1553, -40.5178) (-2.1593, -40.4519) (-2.1747, -40.39) (-2.1723, -40.3199) (-2.2084, -40.263) knots 0 0 0 0 0 1 1 1 1 1
  spline S200 degree 2 poles (2.4585, -43.11) (1.9028, -41.8893) (1.7059, -40.5392) knots 0 0 0 1 1 1
  spline S201 degree 2 poles (-0.4045, -43.1781) (0.0925, -41.9324) (0.225, -40.5744) knots 0 0 0 1 1 1
  spline S202 degree 4 poles (0.225, -40.5744) (0.2321, -40.5088) (0.2504, -40.4478) (0.2514, -40.3776) (0.2901, -40.3225) knots 0 0 0 0 0 1 1 1 1 1
  arc A106 (0.2901, -40.3225) -> (0.9596, -40.3121) centre (0, 0) ccw
  arc A107 (0.9596, -40.3121) -> (1.6288, -40.2906) centre (0, 0) ccw
  spline S203 degree 4 poles (1.7059, -40.5392) (1.6957, -40.4739) (1.6745, -40.4139) (1.6702, -40.3438) (1.6288, -40.2906) knots 0 0 0 0 0 1 1 1 1 1
  spline S204 degree 2 poles (6.5452, -42.6811) (5.8761, -41.5188) (5.5517, -40.1935) knots 0 0 0 1 1 1
  spline S205 degree 2 poles (3.7017, -43.021) (4.078, -41.7338) (4.0808, -40.3693) knots 0 0 0 1 1 1
  spline S206 degree 4 poles (4.0808, -40.3693) (4.0816, -40.3033) (4.094, -40.2408) (4.0883, -40.1709) (4.1217, -40.1123) knots 0 0 0 0 0 1 1 1 1 1
  arc A108 (4.1217, -40.1123) -> (4.7872, -40.0384) centre (0, 0) ccw
  arc A109 (4.7872, -40.0384) -> (5.4513, -39.9534) centre (0, 0) ccw
  spline S207 degree 4 poles (5.5517, -40.1935) (5.5353, -40.1295) (5.5085, -40.0717) (5.4975, -40.0024) (5.4513, -39.9534) knots 0 0 0 0 0 1 1 1 1 1
  spline S208 degree 2 poles (10.5727, -41.8656) (9.7961, -40.7722) (9.3471, -39.4838) knots 0 0 0 1 1 1
  spline S209 degree 2 poles (7.7743, -42.4744) (8.0266, -41.1571) (7.8997, -39.7986) knots 0 0 0 1 1 1
  spline S210 degree 4 poles (7.8997, -39.7986) (7.8942, -39.7328) (7.9006, -39.6694) (7.8883, -39.6003) (7.916, -39.5389) knots 0 0 0 0 0 1 1 1 1 1
  arc A110 (7.916, -39.5389) -> (8.5714, -39.402) centre (0, 0) ccw
  arc A111 (8.5714, -39.402) -> (9.2244, -39.2543) centre (0, 0) ccw
  spline S211 degree 4 poles (9.3471, -39.4838) (9.3248, -39.4216) (9.2926, -39.3666) (9.2751, -39.2987) (9.2244, -39.2543) knots 0 0 0 0 0 1 1 1 1 1
  spline S212 degree 2 poles (14.5044, -40.6711) (13.6274, -39.6564) (13.058, -38.4165) knots 0 0 0 1 1 1
  spline S213 degree 2 poles (11.7766, -41.543) (11.9025, -40.2078) (11.647, -38.8675) knots 0 0 0 1 1 1
  spline S214 degree 4 poles (11.647, -38.8675) (11.6353, -38.8025) (11.6357, -38.7388) (11.6169, -38.6712) (11.6385, -38.6074) knots 0 0 0 0 0 1 1 1 1 1
  arc A112 (11.6385, -38.6074) -> (12.278, -38.4088) centre (0, 0) ccw
  arc A113 (12.278, -38.4088) -> (12.914, -38.1997) centre (0, 0) ccw
  spline S215 degree 4 poles (13.058, -38.4165) (13.0298, -38.3567) (12.9926, -38.305) (12.9687, -38.2391) (12.914, -38.1997) knots 0 0 0 0 0 1 1 1 1 1
  spline S216 degree 2 poles (18.3048, -39.1082) (17.3352, -38.1815) (16.6506, -37.0013) knots 0 0 0 1 1 1
  spline S217 degree 2 poles (15.6722, -40.2355) (15.6706, -38.8943) (15.2889, -37.5844) knots 0 0 0 1 1 1
  spline S218 degree 4 poles (15.2889, -37.5844) (15.271, -37.5208) (15.2653, -37.4574) (15.2402, -37.3918) (15.2557, -37.3263) knots 0 0 0 0 0 1 1 1 1 1
  arc A114 (15.2557, -37.3263) -> (15.8734, -37.0678) centre (0, 0) ccw
  arc A115 (15.8734, -37.0678) -> (16.4867, -36.7992) centre (0, 0) ccw
  spline S219 degree 4 poles (16.6506, -37.0013) (16.6169, -36.9445) (16.5749, -36.8966) (16.5448, -36.8332) (16.4867, -36.7992) knots 0 0 0 0 0 1 1 1 1 1
  spline S220 degree 2 poles (21.9393, -37.1911) (20.8861, -36.3608) (20.0924, -35.251) knots 0 0 0 1 1 1
  spline S221 degree 2 poles (19.4258, -38.5636) (19.2967, -37.2286) (18.7923, -35.9609) knots 0 0 0 1 1 1
  spline S222 degree 4 poles (18.7923, -35.9609) (18.7685, -35.8993) (18.7568, -35.8367) (18.7255, -35.7739) (18.7347, -35.7071) knots 0 0 0 0 0 1 1 1 1 1
  arc A116 (18.7347, -35.7071) -> (19.325, -35.3911) centre (0, 0) ccw
  arc A117 (19.325, -35.3911) -> (19.91, -35.0654) centre (0, 0) ccw
  spline S223 degree 4 poles (20.0924, -35.251) (20.0534, -35.1977) (20.0071, -35.154) (19.9711, -35.0937) (19.91, -35.0654) knots 0 0 0 0 0 1 1 1 1 1
  spline S224 degree 2 poles (25.3752, -34.9372) (24.2479, -34.2108) (23.3522, -33.1815) knots 0 0 0 1 1 1
  spline S225 degree 2 poles (23.0036, -36.5424) (22.7482, -35.2258) (22.1255, -34.0118) knots 0 0 0 1 1 1
  spline S226 degree 4 poles (22.1255, -34.0118) (22.0959, -33.9527) (22.0783, -33.8915) (22.0412, -33.8319) (22.0441, -33.7646) knots 0 0 0 0 0 1 1 1 1 1
  arc A118 (22.0441, -33.7646) -> (22.6017, -33.3939) centre (0, 0) ccw
  arc A119 (22.6017, -33.3939) -> (23.153, -33.014) centre (0, 0) ccw
  spline S227 degree 4 poles (23.3522, -33.1815) (23.3084, -33.1321) (23.2581, -33.093) (23.2166, -33.0364) (23.153, -33.014) knots 0 0 0 0 0 1 1 1 1 1
  spline S228 degree 2 poles (28.5813, -32.367) (27.39, -31.751) (26.4006, -30.8115) knots 0 0 0 1 1 1
  spline S229 degree 2 poles (26.373, -34.1903) (25.9936, -32.9039) (25.2583, -31.7546) knots 0 0 0 1 1 1
  spline S230 degree 4 poles (25.2583, -31.7546) (25.2233, -31.6986) (25.1999, -31.6393) (25.1573, -31.5836) (25.1538, -31.5163) knots 0 0 0 0 0 1 1 1 1 1
  arc A120 (25.1538, -31.5163) -> (25.6736, -31.0943) centre (0, 0) ccw
  arc A121 (25.6736, -31.0943) -> (26.1864, -30.6637) centre (0, 0) ccw
  spline S231 degree 4 poles (26.4006, -30.8115) (26.3522, -30.7665) (26.2984, -30.7323) (26.2517, -30.6799) (26.1864, -30.6637) knots 0 0 0 0 0 1 1 1 1 1
  spline S232 degree 2 poles (31.5286, -29.5036) (30.2841, -29.0036) (29.2099, -28.1624) knots 0 0 0 1 1 1
  spline S233 degree 2 poles (29.5036, -31.5286) (29.0036, -30.2841) (28.1624, -29.2099) knots 0 0 0 1 1 1
  spline S234 degree 4 poles (28.1624, -29.2099) (28.1222, -29.1574) (28.0933, -29.1007) (28.0456, -29.0492) (28.0357, -28.9825) knots 0 0 0 0 0 1 1 1 1 1
  arc A122 (28.0357, -28.9825) -> (28.5131, -28.5131) centre (0, 0) ccw
  arc A123 (28.5131, -28.5131) -> (28.9825, -28.0357) centre (0, 0) ccw
  spline S235 degree 4 poles (29.2099, -28.1624) (29.1574, -28.1222) (29.1007, -28.0933) (29.0492, -28.0456) (28.9825, -28.0357) knots 0 0 0 0 0 1 1 1 1 1
  spline S236 degree 2 poles (34.1903, -26.373) (32.9039, -25.9936) (31.7546, -25.2583) knots 0 0 0 1 1 1
  spline S237 degree 2 poles (32.367, -28.5813) (31.751, -27.39) (30.8115, -26.4006) knots 0 0 0 1 1 1
  spline S238 degree 4 poles (30.8115, -26.4006) (30.7665, -26.3522) (30.7323, -26.2984) (30.6799, -26.2517) (30.6637, -26.1864) knots 0 0 0 0 0 1 1 1 1 1
  arc A124 (30.6637, -26.1864) -> (31.0943, -25.6736) centre (0, 0) ccw
  arc A125 (31.0943, -25.6736) -> (31.5163, -25.1538) centre (0, 0) ccw
  spline S239 degree 4 poles (31.7546, -25.2583) (31.6986, -25.2233) (31.6393, -25.1999) (31.5836, -25.1573) (31.5163, -25.1538) knots 0 0 0 0 0 1 1 1 1 1
  spline S240 degree 2 poles (36.5424, -23.0036) (35.2258, -22.7482) (34.0118, -22.1255) knots 0 0 0 1 1 1
  spline S241 degree 2 poles (34.9372, -25.3752) (34.2108, -24.2479) (33.1815, -23.3522) knots 0 0 0 1 1 1
  spline S242 degree 4 poles (33.1815, -23.3522) (33.1321, -23.3084) (33.093, -23.2581) (33.0364, -23.2166) (33.014, -23.153) knots 0 0 0 0 0 1 1 1 1 1
  arc A126 (33.014, -23.153) -> (33.3939, -22.6017) centre (0, 0) ccw
  arc A127 (33.3939, -22.6017) -> (33.7646, -22.0441) centre (0, 0) ccw
  spline S243 degree 4 poles (34.0118, -22.1255) (33.9527, -22.0959) (33.8915, -22.0783) (33.8319, -22.0412) (33.7646, -22.0441) knots 0 0 0 0 0 1 1 1 1 1
  spline S244 degree 2 poles (38.5636, -19.4258) (37.2286, -19.2967) (35.9609, -18.7923) knots 0 0 0 1 1 1
  spline S245 degree 2 poles (37.1911, -21.9393) (36.3608, -20.8861) (35.251, -20.0924) knots 0 0 0 1 1 1
  spline S246 degree 4 poles (35.251, -20.0924) (35.1977, -20.0534) (35.154, -20.0071) (35.0937, -19.9711) (35.0654, -19.91) knots 0 0 0 0 0 1 1 1 1 1
  arc A128 (35.0654, -19.91) -> (35.3911, -19.325) centre (0, 0) ccw
  arc A129 (35.3911, -19.325) -> (35.7071, -18.7347) centre (0, 0) ccw
  spline S247 degree 4 poles (35.9609, -18.7923) (35.8993, -18.7685) (35.8367, -18.7568) (35.7739, -18.7255) (35.7071, -18.7347) knots 0 0 0 0 0 1 1 1 1 1
  spline S248 degree 2 poles (40.2355, -15.6722) (38.8943, -15.6706) (37.5844, -15.2889) knots 0 0 0 1 1 1
  spline S249 degree 2 poles (39.1082, -18.3048) (38.1815, -17.3352) (37.0013, -16.6506) knots 0 0 0 1 1 1
  spline S250 degree 4 poles (37.0013, -16.6506) (36.9445, -16.6169) (36.8966, -16.5749) (36.8332, -16.5448) (36.7992, -16.4867) knots 0 0 0 0 0 1 1 1 1 1
  arc A130 (36.7992, -16.4867) -> (37.0678, -15.8734) centre (0, 0) ccw
  arc A131 (37.0678, -15.8734) -> (37.3263, -15.2557) centre (0, 0) ccw
  spline S251 degree 4 poles (37.5844, -15.2889) (37.5208, -15.271) (37.4574, -15.2653) (37.3918, -15.2402) (37.3263, -15.2557) knots 0 0 0 0 0 1 1 1 1 1
  spline S252 degree 2 poles (41.543, -11.7766) (40.2078, -11.9025) (38.8675, -11.647) knots 0 0 0 1 1 1
  spline S253 degree 2 poles (40.6711, -14.5044) (39.6564, -13.6274) (38.4165, -13.058) knots 0 0 0 1 1 1
  spline S254 degree 4 poles (38.4165, -13.058) (38.3567, -13.0298) (38.305, -12.9926) (38.2391, -12.9687) (38.1997, -12.914) knots 0 0 0 0 0 1 1 1 1 1
  arc A132 (38.1997, -12.914) -> (38.4088, -12.278) centre (0, 0) ccw
  arc A133 (38.4088, -12.278) -> (38.6074, -11.6385) centre (0, 0) ccw
  spline S255 degree 4 poles (38.8675, -11.647) (38.8025, -11.6353) (38.7388, -11.6357) (38.6712, -11.6169) (38.6074, -11.6385) knots 0 0 0 0 0 1 1 1 1 1
  spline S256 degree 2 poles (42.4744, -7.7743) (41.1571, -8.0266) (39.7986, -7.8997) knots 0 0 0 1 1 1
  spline S257 degree 2 poles (41.8656, -10.5727) (40.7722, -9.7961) (39.4838, -9.3471) knots 0 0 0 1 1 1
  spline S258 degree 4 poles (39.4838, -9.3471) (39.4216, -9.3248) (39.3666, -9.2926) (39.2987, -9.2751) (39.2543, -9.2244) knots 0 0 0 0 0 1 1 1 1 1
  arc A134 (39.2543, -9.2244) -> (39.402, -8.5714) centre (0, 0) ccw
  arc A135 (39.402, -8.5714) -> (39.5389, -7.916) centre (0, 0) ccw
  spline S259 degree 4 poles (39.7986, -7.8997) (39.7328, -7.8942) (39.6694, -7.9006) (39.6003, -7.8883) (39.5389, -7.916) knots 0 0 0 0 0 1 1 1 1 1
  spline S260 degree 2 poles (43.021, -3.7017) (41.7338, -4.078) (40.3693, -4.0808) knots 0 0 0 1 1 1
  spline S261 degree 2 poles (42.6811, -6.5452) (41.5188, -5.8761) (40.1935, -5.5517) knots 0 0 0 1 1 1
  spline S262 degree 4 poles (40.1935, -5.5517) (40.1295, -5.5353) (40.0717, -5.5085) (40.0024, -5.4975) (39.9534, -5.4513) knots 0 0 0 0 0 1 1 1 1 1
  arc A136 (39.9534, -5.4513) -> (40.0384, -4.7872) centre (0, 0) ccw
  arc A137 (40.0384, -4.7872) -> (40.1123, -4.1217) centre (0, 0) ccw
  spline S263 degree 4 poles (40.3693, -4.0808) (40.3033, -4.0816) (40.2408, -4.094) (40.1709, -4.0883) (40.1123, -4.1217) knots 0 0 0 0 0 1 1 1 1 1
  point P0 (41.8625, -1.9942)
  point P1 (40.4117, -1.6779)
  point P2 (40.4752, -1.693)
  point P3 (40.3487, -1.6594)
  point P4 (41.7202, 3.9838)
  point P5 (41.8625, 1.9942)
  point P6 (40.4528, 2.1621)
  point P7 (40.3882, 2.1711)
  point P8 (40.3237, 2.1835)
  point P9 (40.2208, 2.8766)
  point P10 (40.3488, 3.617)
  point P11 (40.286, 3.5988)
  point P12 (40.224, 3.5774)
  point P13 (41.1526, 7.9315)
  point P14 (41.4834, 5.9644)
  point P15 (40.0641, 5.9976)
  point P16 (39.9989, 6.0004)
  point P17 (39.9336, 6.0067)
  point P18 (39.8223, 7.436)
  point P19 (39.7615, 7.412)
  point P20 (39.7019, 7.3847)
  point P21 (40.2124, 11.8074)
  point P22 (40.7286, 9.8807)
  point P23 (39.3126, 9.7787)
  point P24 (39.2474, 9.7754)
  point P25 (39.1818, 9.7754)
  point P26 (38.9351, 11.1877)
  point P27 (38.8769, 11.158)
  point P28 (38.8201, 11.1252)
  point P29 (38.9079, 15.5764)
  point P30 (39.605, 13.7074)
  point P31 (38.2051, 13.4714)
  point P32 (38.1405, 13.4618)
  point P33 (38.0752, 13.4556)
  point P34 (37.7811, 14.0916)
  point P35 (37.6953, 14.838)
  point P36 (37.6403, 14.8029)
  point P37 (37.5868, 14.7649)
  point P38 (37.2511, 19.2043)
  point P39 (38.1227, 17.41)
  point P40 (36.7515, 17.042)
  point P41 (36.6882, 17.0263)
  point P42 (36.6237, 17.0139)
  point P43 (36.2706, 17.6192)
  point P44 (36.1142, 18.354)
  point P45 (36.0627, 18.3138)
  point P46 (36.0131, 18.2709)
  point P47 (35.2569, 22.6583)
  point P48 (36.2951, 20.955)
  point P49 (34.9652, 20.4583)
  point P50 (34.9036, 20.4367)
  point P51 (34.8406, 20.4182)
  point P52 (34.4315, 20.9871)
  point P53 (34.206, 21.7038)
  point P54 (34.1586, 21.6589)
  point P55 (34.1133, 21.6114)
  point P56 (32.9435, 25.907)
  point P57 (34.1389, 24.3102)
  point P58 (32.8622, 23.6893)
  point P59 (32.8029, 23.6619)
  point P60 (32.742, 23.6376)
  point P61 (31.9881, 24.857)
  point P62 (31.9451, 24.8078)
  point P63 (31.9046, 24.7562)
  point P64 (30.3317, 28.9212)
  point P65 (31.6735, 27.4452)
  point P66 (30.4616, 26.7058)
  point P67 (30.4051, 26.6729)
  point P68 (30.3468, 26.6429)
  point P69 (29.4804, 27.7851)
  point P70 (29.4423, 27.732)
  point P71 (29.4069, 27.6768)
  point P72 (27.4452, 31.6735)
  point P73 (28.9212, 30.3317)
  point P74 (27.7851, 29.4804)
  point P75 (27.732, 29.4423)
  point P76 (27.6768, 29.4069)
  point P77 (27.1241, 29.8375)
  point P78 (26.7058, 30.4616)
  point P79 (26.6729, 30.4051)
  point P80 (26.6429, 30.3468)
  point P81 (24.3102, 34.1389)
  point P82 (25.907, 32.9435)
  point P83 (24.857, 31.9881)
  point P84 (24.8078, 31.9451)
  point P85 (24.7562, 31.9046)
  point P86 (24.165, 32.2807)
  point P87 (23.6893, 32.8622)
  point P88 (23.6619, 32.8029)
  point P89 (23.6376, 32.742)
  point P90 (20.955, 36.2951)
  point P91 (22.6583, 35.2569)
  point P92 (21.7038, 34.206)
  point P93 (21.6589, 34.1586)
  point P94 (21.6114, 34.1133)
  point P95 (20.4583, 34.9652)
  point P96 (20.4367, 34.9036)
  point P97 (20.4182, 34.8406)
  point P98 (17.41, 38.1227)
  point P99 (19.2043, 37.2511)
  point P100 (18.354, 36.1142)
  point P101 (18.3138, 36.0627)
  point P102 (18.2709, 36.0131)
  point P103 (17.6192, 36.2706)
  point P104 (17.042, 36.7515)
  point P105 (17.0263, 36.6882)
  point P106 (17.0139, 36.6237)
  point P107 (13.7074, 39.605)
  point P108 (15.5764, 38.9079)
  point P109 (14.838, 37.6953)
  point P110 (14.8029, 37.6403)
  point P111 (14.7649, 37.5868)
  point P112 (14.0916, 37.7811)
  point P113 (13.4714, 38.2051)
  point P114 (13.4618, 38.1405)
  point P115 (13.4556, 38.0752)
  point P116 (9.8807, 40.7286)
  point P117 (11.8074, 40.2124)
  point P118 (11.1877, 38.9351)
  point P119 (11.158, 38.8769)
  point P120 (11.1252, 38.8201)
  point P121 (10.4365, 38.9496)
  point P122 (9.7787, 39.3126)
  point P123 (9.7754, 39.2474)
  point P124 (9.7754, 39.1818)
  point P125 (5.9644, 41.4834)
  point P126 (7.9315, 41.1526)
  point P127 (7.436, 39.8223)
  point P128 (7.412, 39.7615)
  point P129 (7.3847, 39.7019)
  point P130 (6.6869, 39.7652)
  point P131 (5.9976, 40.0641)
  point P132 (6.0004, 39.9989)
  point P133 (6.0067, 39.9336)
  point P134 (1.9942, 41.8625)
  point P135 (3.9838, 41.7202)
  point P136 (3.617, 40.3488)
  point P137 (3.5988, 40.286)
  point P138 (3.5774, 40.224)
  point P139 (2.8766, 40.2208)
  point P140 (2.1621, 40.4528)
  point P141 (2.1711, 40.3882)
  point P142 (2.1835, 40.3237)
  point P143 (-1.9942, 41.8625)
  point P144 (0, 41.91)
  point P145 (-0.2348, 40.5099)
  point P146 (-0.2469, 40.4457)
  point P147 (-0.2624, 40.382)
  point P148 (-0.9596, 40.3121)